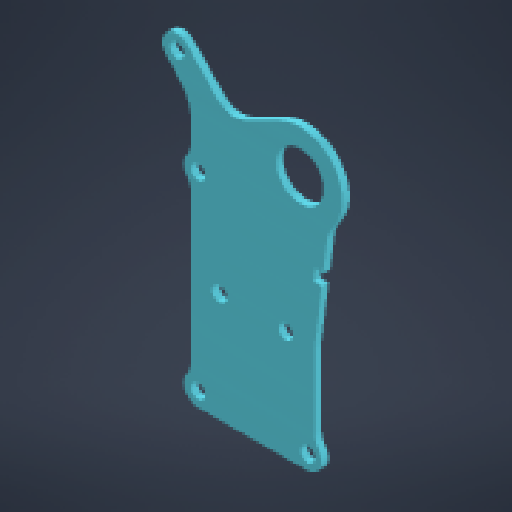
# Autodesk Inventor part: tibea_outside_steel
Saved by Autodesk Inventor 2026 (Build 300175000, 175)
## iProperties
Created: 2026-04-23
Part Number: tibea_outside_steel
Material: Сталь
Document SubType Name: Modeling
Designer: user
Density: 7.85 g/cm^3
Appearance: Серо-синий
Mass: 156.465 g
Surface Area: 150.385 cm^2
Volume: 19.9318 cm^3
Author: user
Autodesk Inventor part; units mm, degrees
ref_plane "YZ Plane" through (0, 0, 0) normal (1, 0, 0) x (0, 1, 0)
ref_plane "XZ Plane" through (0, 0, 0) normal (0, 1, 0) x (-1, 0, 0)
ref_plane "XY Plane" through (0, 0, 0) normal (0, 0, 1) x (1, 0, 0)
sketch "Эскиз1" plane through (0, 0, 0) normal (0, 0, 1) x (1, 0, 0)
  line L0 (-302.1837, 10.5492) -> (-302.1837, 17.7522) construction
  line L1 (-302.1837, 21.7824) -> (-325.2337, 21.7824)
  circle A0 centre (-325.2337, 27.8824) radius 3.05
  arc A1 (-330.1781, 31.4549) -> (-325.2337, 21.7824) centre (-325.2337, 27.8824) ccw
  circle A2 centre (-316.1337, 67.8824) radius 3.05
  line L2 (-328.2837, 37.3115) -> (-328.2837, 98.4533)
  arc A3 (-330.1781, 111.4549) -> (-330.1781, 104.3099) centre (-325.2337, 107.8824) ccw
  circle A4 centre (-325.2337, 107.8824) radius 3.05
  line L3 (-302.1837, 21.7824) -> (-279.1337, 21.7824)
  circle A5 centre (-279.1337, 27.8824) radius 3.05
  arc A6 (-279.1337, 21.7824) -> (-274.1893, 31.4549) centre (-279.1337, 27.8824) ccw
  circle A7 centre (-288.2337, 67.8824) radius 3.05
  line L4 (-276.0837, 37.3115) -> (-276.0837, 55.2722)
  circle A8 centre (-282.1837, 127.8824) radius 10.05
  circle A9 centre (-334.1837, 147.8824) radius 3.05
  arc A10 (-328.2837, 98.4533) -> (-330.1781, 104.3099) centre (-338.2837, 98.4533) ccw
  arc A11 (-276.0837, 37.3115) -> (-274.1893, 31.4549) centre (-266.0837, 37.3115) ccw
  arc A12 (-330.1781, 31.4549) -> (-328.2837, 37.3115) centre (-338.2837, 37.3115) ccw
  arc A13 (-265.5872, 116.722) -> (-290.9228, 145.8721) centre (-282.1837, 127.8824) ccw
  line L5 (-338.6099, 136.8725) -> (-338.5459, 136.8362)
  line L6 (-328.2837, 117.3115) -> (-328.2837, 124.794)
  arc A14 (-330.1781, 111.4549) -> (-328.2837, 117.3115) centre (-338.2837, 117.3115) ccw
  line L7 (-276.5228, 92.4146) -> (-271.562, 91.7896)
  line L8 (-275.8853, 97.4746) -> (-270.9245, 96.8496)
  line L9 (-275.8853, 97.4746) -> (-276.5228, 92.4146)
  arc A15 (-265.5872, 116.722) -> (-268.3702, 112.0542) centre (-224.0958, 88.8209) ccw
  line L10 (-276.0053, 56.5222) -> (-271.562, 91.7896)
  line L11 (-270.9245, 96.8496) -> (-269.4369, 108.6576)
  arc A16 (-268.3702, 112.0542) -> (-269.4369, 108.6576) centre (-259.5153, 107.4076) ccw
  arc A17 (-276.0053, 56.5222) -> (-276.0837, 55.2722) centre (-266.0837, 55.2722) ccw
  line L12 (-329.7466, 152.0683) -> (-318.576, 140.2274) construction
  arc A18 (-329.7466, 152.0683) -> (-338.6208, 143.6964) centre (-334.1837, 147.8824) ccw
  line L13 (-306.9325, 138.0948) -> (-290.9228, 145.8721)
  line L14 (-318.576, 140.2274) -> (-329.7466, 152.0683)
  arc A19 (-318.576, 140.2274) -> (-306.9325, 138.0948) centre (-311.302, 147.0897) ccw
  line L15 (-338.6208, 143.6964) -> (-333.7359, 138.5184)
  arc A20 (-328.2837, 124.794) -> (-333.7359, 138.5184) centre (-348.2837, 124.794) ccw
  point P0 (-328.2837, 33.1651)
  point P1 (-328.2837, 102.5996)
  point P2 (-276.0837, 33.1651)
  point P3 (-273.9038, 109.6768)
  point P4 (-331.3337, 107.8824)
  point P5 (-276.0837, 108.8353)
  point P6 (-274.0504, 146.1539)
  point P7 (-328.2837, 163.1651)
  point P8 (-292.0449, 110.4825)
  point P9 (-328.2837, 113.1651)
  point P10 (-274.0806, 92.107)
  point P11 (-273.2011, 97.1365)
  point P12 (-274.0056, 92.0975)
  point P13 (-269.2237, 110.3494)
  dimension "d0" = 6.1
  dimension "d1" = 12.2
  dimension "d2" = 46.1
  dimension "d10" = 80
  dimension "d11" = 40
  dimension "d12" = 9.1
  dimension "d13" = 20.1
  dimension "d15" = 60
  dimension "d17" = 20
  dimension "d23" = 40
  dimension "d31" = 10
  dimension "d35" = 5.1
  dimension "d37" = 50
  dimension "d41" = 18
  dimension "d42" = 12.2
  dimension "d43" = 52
  dimension "d44" = 20
  dimension "d45" = 10
  dimension "d46" = 20
  dimension "d47" = 5
  constraints: 38 point on circle, 32 end point, 24 tangent, 21 centre point, 12 point on line, 9 equal radius, 5 coincident, 5 symmetric about line, 4 vertical, 2 perpendicular, 2 vertical alignment, 1 collinear, 1 horizontal, 1 parallel, 5 other
  measures "d0" diameter of A0
  measures "d1" diameter of A1
  measures "d2" diameter of A0.centre L0
  measures "d10" distance of A3.centre A0.centre
  measures "d11" vertical distance of A0.centre A2.centre
  measures "d12" horizontal distance of A2.centre A0.centre
  measures "d13" diameter of A8
  measures "d15" vertical distance of A8.centre A7.centre
  measures "d17" distance from line of L0 A8.centre
  measures "d23" diameter of A13
  measures "d31" radius of A14
  measures "d35" distance from line of L8 point (-274.006, 92.098)
  measures "d37" radius of A15
  measures "d41" distance from line of A8.centre L12
  measures "d42" diameter of A18
  measures "d43" horizontal distance of A9.centre A8.centre
  measures "d44" vertical distance of A9.centre A8.centre
  measures "d45" radius of A19
  measures "d46" radius of A20
  measures "d47" distance between parallel lines of L11 L9
extrude "Выдавливание1" add sketch "Эскиз1" along normal blind 3
equation "\"d0\" = d_main_screw_holes"
equation "\"d1\" = 2 * d_main_screw_holes"
equation "\"d2\" = hight_profile_tibea + d_main_screw_holes"
equation "\"d12\" = d_main_screw_holes + thickness_profile_tibea"
equation "\"d21\" = thickness_steel"
equation "\"tolerance_plazma\" = 0.1"
equation "\"thickness_steel\" = 3"
equation "\"d_main_screw_holes\" = 6.1"
equation "\"thickness_profile_tibea\" = 3"
equation "\"hight_profile_tibea\" = 40"
equation "\"hight_shaft_shift\" = 37"
equation "\"thickness_profile_femur\" = 3"
equation "\"width_shaft_shift\" = 35"
equation "\"width_flattened_surface\" = 12"
